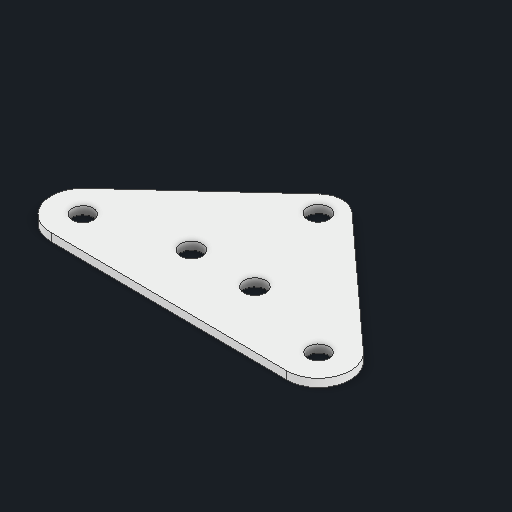
# Autodesk Inventor part: MOGO Clamp Gusset
Saved by Autodesk Inventor 2025.1 (Build 291241000, 241)
## iProperties
Created: 2024-11-26
Part Number: MOGO Clamp Gusset
Material: Acetal Resin, White
Document SubType Name: Modeling
Designer: avere
Density: 1.425 g/cm^3
Appearance: Smooth - White
Author: avere
Autodesk Inventor part; units mm, degrees
ref_plane "YZ Plane" through (0, 0, 0) normal (1, 0, 0) x (0, 1, 0)
ref_plane "XZ Plane" through (0, 0, 0) normal (0, 1, 0) x (-1, 0, 0)
ref_plane "XY Plane" through (0, 0, 0) normal (0, 0, 1) x (1, 0, 0)
sketch "Sketch1" plane through (0, 0, 0) normal (0, 1, 0) x (-1, 0, 0)
  circle A0 centre (5.98, -1.0093) radius 2.1844
  circle A1 centre (-6.72, -1.0093) radius 2.1844
  arc A2 (25.9781, -1.9806) -> (23.0279, 9.9925) centre (23.0279, 3.6425) ccw
  arc A3 (-24.4341, 10.3681) -> (-27.4345, -1.6047) centre (-24.4843, 4.0183) ccw
  circle A4 centre (23.0279, 3.6425) radius 2.0955
  circle A5 centre (-24.4843, 4.0183) radius 2.0955
  line L0 (23.0279, 9.9925) -> (-24.4341, 10.3681)
  circle A6 centre (-0.37, -20.0593) radius 2.1844
  arc A7 (-3.5744, -23.5826) -> (2.8559, -23.5628) centre (-0.37, -20.0593) ccw
  line L1 (27.3291, -1.0289) -> (2.8559, -23.5628)
  line L2 (-28.7568, -0.6794) -> (-3.5744, -23.5826)
  point P0 (0, 0)
  dimension "d0" = 12.7
  dimension "d1" = 12.7
  dimension "d2" = 4.191
  dimension "d3" = 4.191
  dimension "d4" = 9.525
  constraints: 8 centre point, 8 point on circle, 6 end point, 5 tangent, 3 coincident
  measures "d0" diameter of A2
  measures "d1" diameter of A3
  measures "d2" diameter of A4
  measures "d3" diameter of A5
  measures "d4" diameter of A7
extrude "Extrusion1" add sketch "Sketch1" along normal blind 1.5875
body "Solid1"
